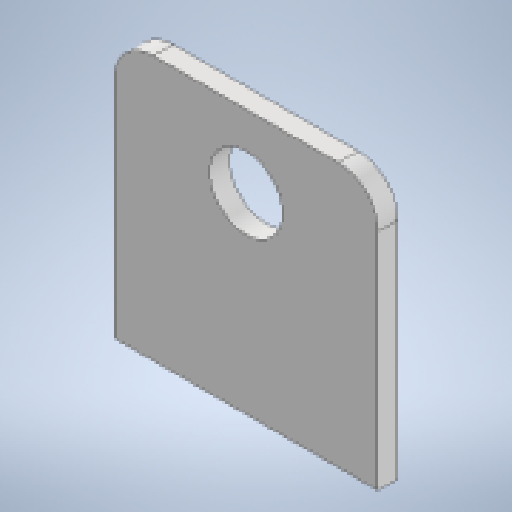
# Autodesk Inventor part: ДМФ 094 Постель НОС крепление v2.0
Saved by Autodesk Inventor 2026.2 (Build 302298000, 298)
## iProperties
Created: 2024-04-28
Part Number: ДМФ 094 Постель НОС крепление v2.0
Material: Generic
Document SubType Name: Sheet Metal
Designer: pokla
Stock Number: Постель_Нос
Density: 1 g/cm^3
Sheet Metal Rule: Default
Sheet Metal Width: 0,000 mm
Sheet Metal Length: 0,000 mm
Sheet Metal Area: 0,000 mm^2
Appearance: Default
Author: pokla
Autodesk Inventor part; units mm, degrees
ref_plane "YZ Plane" through (0, 0, 0) normal (1, 0, 0) x (0, 1, 0)
ref_plane "XZ Plane" through (0, 0, 0) normal (0, 1, 0) x (-1, 0, 0)
ref_plane "XY Plane" through (0, 0, 0) normal (0, 0, 1) x (1, 0, 0)
sketch "Sketch12" plane through (0, 0, 0) normal (0, 0, 1) x (1, 0, 0)
  line L0 (-20, 26) -> (20, 26)
  line L1 (20, 26) -> (20, 0)
  line L2 (20, 0) -> (-20, 0)
  line L3 (-20, 0) -> (-20, 26)
  circle A0 centre (0, 15) radius 5.5
  point P0 (0, 0)
  point P1 (0, 0)
  dimension "d73" = 40
  dimension "d74" = 11
  dimension "d77" = 15
  dimension "d78" = 26
  measures "d73" distance of L1.end L2.end
  measures "d74" diameter of A0
  measures "d77" distance of A0.centre point (0, 0)
  measures "d78" distance of L0.end L1.end
extrude "Plate3" add sketch "Sketch12" along normal blind 3
fillet "Corner Round1" radius 6 2 edges at (-20, 26, 1.5) (20, 26, 1.5)
equation "\"d75\" = Thickness"
equation "\"BendRadius\" = Thickness"
equation "\"BendReliefWidth\" = Thickness"
equation "\"BendReliefDepth\" = 0.5 * Thickness"
equation "\"CornerReliefSize\" = 4 * Thickness"
equation "\"MinimumRemnant\" = 2 * Thickness"
equation "\"TransitionRadius\" = BendRadius"
equation "\"JacobiRadiusSize\" = BendRadius"
equation "\"GapSize\" = Thickness"
equation "\"Thickness\" = 3"
body "Solid4"
